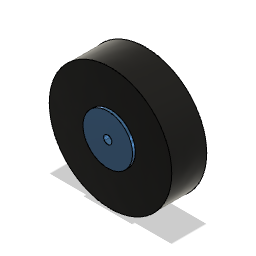
_fingertech 1.75 x .603ab60a-0eeb-4a23-a273-b403b345e76f (Autodesk Fusion 360 design; units mm, degrees)
Autodesk Fusion 360 part; units mm, degrees
sketch "Sketch4" plane through (0, 0, 0) normal (0, 0, 1) x (1, 0, 0)
  circle A0 centre (0, 0) radius 22.225
  circle A1 centre (0, 0) radius 5
  circle A2 centre (0, 0) radius 1.5
  circle A3 centre (0, 0) radius 9
  dimension "d64" = 44.45
  dimension "d65" = 10
  dimension "d66" = 3
  dimension "d71" = 18
  constraint coincident A0.centre A1.centre
  constraint concentric A0 A1
  constraint concentric A0 A2
  measures "d64" diameter of A0
  measures "d65" diameter of A1
  measures "d66" diameter of A2
  measures "d71" diameter of A3
extrude "Extrude7" add sketch "Sketch4" against normal blind 1 contours A1 | A3 makes body 1
extrude "Extrude5" add sketch "Sketch4" along normal blind 12.7 separate body contours A0 | A3 makes body 2
extrude "Extrude6" add sketch "Sketch4" along normal blind 12.7 separate body contours A1 makes body 3
copy_body "CopyPasteBodies1" bodies 1 makes body 4
move_body "Move1" bodies 4 to x (1, 0, 0) y (0, 1, 0) z (0, 0, 1) at (0, 0, 13.7)
combine "Combine1" operation add target body 4 tool bodies 3 1
named bodies: "wheel", "hub"
